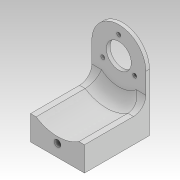
# Autodesk Inventor part: TestEncoderBracket
Saved by Autodesk Inventor 2020 (Build 240168000, 168)
## iProperties
Created: 2022-01-16
Part Number: TestEncoderBracket
Material: Generic
Document SubType Name: Modeling
Designer: DDeGo
Density: 1 g/cm^3
Appearance: Default
Author: DDeGo
Autodesk Inventor part; units mm, degrees
ref_plane "YZ Plane" through (0, 0, 0) normal (1, 0, 0) x (0, 1, 0)
ref_plane "XZ Plane" through (0, 0, 0) normal (0, 1, 0) x (-1, 0, 0)
ref_plane "XY Plane" through (0, 0, 0) normal (0, 0, 1) x (1, 0, 0)
sketch "Sketch1" plane through (0, 0, 0) normal (0, 0, 1) x (1, 0, 0)
  circle A0 centre (0, 0) radius 10.15
  arc A1 (22, 0) -> (-22, 0) centre (0, 0) ccw
  line L0 (-22, 0) -> (22, 0) construction
  line L1 (22, 0) -> (22, -46.826)
  line L2 (22, -46.826) -> (-22, -46.826)
  line L3 (-22, -46.826) -> (-22, 0)
  circle A2 centre (0, 0) radius 15 construction
  circle A3 centre (0, 15) radius 1.6
  line L4 (0, 15) -> (0, 0) construction
  circle A4 centre (-12.9904, -7.5) radius 1.6
  circle A5 centre (12.9904, -7.5) radius 1.6
  dimension "d3" = 30
  dimension "d0" = 20.3
  dimension "d1" = 46.826
  dimension "d2" = 22
  dimension "d4" = 3.2
  dimension "d7" = 360
  constraints: 10 end point, 5 centre point, 3 coincident, 2 parallel, 2 point on circle, 1 horizontal, 1 midpoint, 1 perpendicular, 1 vertical, 1 vertical alignment, 9 other
  measures "d0" diameter of A0
  measures "d1" distance between parallel lines of L2 L0
  measures "d2" radius of A1
  measures "d4" diameter of A3
extrude "Extrusion1" add sketch "Sketch1" along normal blind 3
sketch "Sketch2" plane through (0, 0, 3) normal (0, 0, 1) x (1, 0, 0)
  line L0 (-22, -46.826) -> (22, -46.826) projected
  line L1 (-22, 0) -> (-22, -46.826) projected
  line L2 (22, -46.826) -> (-22, -46.826)
  line L3 (-22, -46.826) -> (-22, -26.826)
  line L4 (22, -26.826) -> (22, -46.826)
  arc A0 (-17.4461, -26.826) -> (17.4461, -26.826) centre (0, 0) ccw
  line L5 (-22, -26.826) -> (-17.4461, -26.826)
  line L6 (17.4461, -26.826) -> (22, -26.826)
  dimension "d14" = 32
  dimension "d15" = 20
  constraints: 10 end point, 3 parallel, 2 point on circle, 1 centre point, 1 coincident, 1 collinear, 1 horizontal, 1 perpendicular, 1 point on line
  measures "d14" radius of A0
  measures "d15" distance between parallel lines of L0 L5
extrude "Extrusion2" add sketch "Sketch2" along normal blind 50
sketch "Sketch3" plane through (0, 0, 53) normal (0, 0, 1) x (1, 0, 0)
  line L0 (-22, -46.826) -> (22, -46.826) projected
  line L1 (0, -46.826) -> (0, -36.826) construction
  circle A0 centre (0, -36.826) radius 2.75
  point P0 (0, 0)
  dimension "d16" = 10
  dimension "d17" = 5.5
  constraints: 2 end point, 1 centre point, 1 coincident, 1 midpoint, 1 vertical
  measures "d16" distance of L1.start L1.end
  measures "d17" diameter of A0
extrude "Extrusion3" cut sketch "Sketch3" against normal through all
sketch "Sketch4" plane through (0, 0, 0) normal (0, 0, -1) x (-1, 0, 0)
  circle A0 centre (0, -36.826) radius 2.75 projected
  circle A1 centre (0, -36.826) radius 4.5
  point P0 (0, 0)
  dimension "d20" = 9
  constraints: 1 centre point, 1 coincident
  measures "d20" diameter of A1
extrude "Extrusion4" cut sketch "Sketch4" against normal blind 24 contours A0 | A1
fillet "Fillet1" radius 10 3 edges at (0, -32, 3) (-19.723, -26.826, 3) (19.723, -26.826, 3)
body "Solid1"
